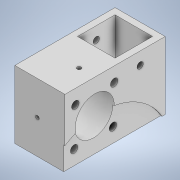
# Autodesk Inventor part: nema_mount
Saved by Autodesk Inventor 2022.3 (Build 263350000, 350)
## iProperties
Created: 2022-06-10
Part Number: nema_mount
Material: Generic
Document SubType Name: Modeling
Designer: Martijn
Density: 1 g/cm^3
Appearance: Default
Author: Martijn
Autodesk Inventor part; units mm, degrees
ref_plane "YZ Plane" through (0, 0, 0) normal (1, 0, 0) x (0, 1, 0)
ref_plane "XZ Plane" through (0, 0, 0) normal (0, 1, 0) x (-1, 0, 0)
ref_plane "XY Plane" through (0, 0, 0) normal (0, 0, 1) x (1, 0, 0)
sketch "Sketch1" plane through (0, 0, 0) normal (0, 0, 1) x (1, 0, 0)
  line L0 (0, 0) -> (40, 0)
  line L1 (40, 0) -> (40, 54)
  line L2 (40, 54) -> (0, 54)
  line L3 (0, 54) -> (0, 0)
  dimension "d0" = 40
  dimension "d1" = 54
  constraints: 8 end point, 2 parallel, 1 horizontal, 1 perpendicular
  measures "d0" distance of L0.start L0.end
  measures "d1" distance of L2.end L0.start
extrude "Extrusion1" add sketch "Sketch1" along normal blind 80
sketch "Sketch3" plane through (0, 0, 0) normal (0, -1, 0) x (1, 0, 0)
  line L0 (5, 5) -> (35, 5)
  line L1 (35, 5) -> (35, 35)
  line L2 (35, 35) -> (5, 35)
  line L3 (5, 35) -> (5, 5)
  line L4 (0, 0) -> (40, 0) projected
  line L5 (0, 0) -> (0, 80) projected
  dimension "d7" = 30
  dimension "d8" = 30
  dimension "d9" = 5
  dimension "d10" = 5
  constraints: 8 end point, 2 parallel, 1 horizontal, 1 perpendicular
  measures "d7" distance between parallel lines of L2 L0
  measures "d8" distance between parallel lines of L1 L3
  measures "d9" distance between parallel lines of L4 L0
  measures "d10" distance between parallel lines of L5 L3
extrude "Extrusion2" cut sketch "Sketch3" against normal blind 80
sketch "Sketch4" plane through (0, 0, 0) normal (-1, 0, 0) x (0, 0, 1)
  line L0 (35, 0) -> (35, 54) projected
  line L1 (35, 5.8) -> (77.4, 5.8)
  line L2 (77.4, 5.8) -> (77.4, 48.2)
  line L3 (77.4, 48.2) -> (35, 48.2)
  line L4 (35, 48.2) -> (35, 5.8)
  line L5 (0, 0) -> (80, 0) projected
  dimension "d13" = 42.4
  dimension "d14" = 42.4
  dimension "d15" = 5.8
  constraints: 8 end point, 2 parallel, 1 horizontal, 1 perpendicular, 1 point on line
  measures "d13" distance between parallel lines of L3 L1
  measures "d14" distance between parallel lines of L0 L2
  measures "d15" distance between parallel lines of L5 L1
extrude "Extrusion3" cut sketch "Sketch4" against normal blind 9
sketch "Sketch5" plane through (9, 0, 0) normal (-1, 0, 0) x (0, 0, 1)
  circle A0 centre (71.7, 42.5) radius 1.6
  circle A1 centre (71.7, 11.5) radius 1.6
  circle A2 centre (40.7, 42.5) radius 1.6
  circle A3 centre (40.7, 11.5) radius 1.6
  circle A4 centre (56.2, 27) radius 2.75
  line L0 (71.7, 42.5) -> (71.7, 11.5)
  line L1 (71.7, 11.5) -> (40.7, 11.5)
  line L2 (40.7, 11.5) -> (40.7, 42.5)
  line L3 (40.7, 42.5) -> (71.7, 42.5)
  line L4 (77.4, 48.2) -> (77.4, 5.8) projected
  line L5 (35, 48.2) -> (77.4, 48.2) projected
  point P0 (0, 0)
  dimension "d18" = 3.2
  dimension "d19" = 31
  dimension "d20" = 31
  dimension "d21" = 5.7
  dimension "d22" = 5.7
  dimension "d23" = 15.5
  dimension "d24" = 15.5
  dimension "d25" = 5.5
  constraints: 8 end point, 5 centre point, 3 equal radius, 3 perpendicular, 1 vertical
  measures "d18" diameter of A0
  measures "d19" distance of L0.start L0.end
  measures "d20" distance of L2.end L0.start
  measures "d21" distance between parallel lines of L4 L0
  measures "d22" distance between parallel lines of L5 L3
  measures "d23" horizontal distance of A4.centre L0.start
  measures "d24" horizontal distance of L2.end A4.centre
  measures "d25" diameter of A4
extrude "Extrusion4" cut sketch "Sketch5" against normal blind 40 contours A0 L0 L3 | L3 L0 A0 | L3 L2 A2 | A2 L2 L3 | L0 L1 A1 | A1 L1 L0 | L2 L1 A3 | A3 L1 L2 | A4
sketch "Sketch7" plane through (40, 0, 0) normal (1, 0, 0) x (0, 0, -1)
  circle A0 centre (-56.2, 27) radius 15.5
  circle A1 centre (-56.2, 27) radius 2.75 projected
  circle A2 centre (-71.7, 11.5) radius 1.6 projected
  circle A3 centre (-71.7, 11.5) radius 3
  circle A4 centre (-40.7, 11.5) radius 1.6 projected
  circle A5 centre (-40.7, 11.5) radius 3
  circle A6 centre (-40.7, 42.5) radius 1.6 projected
  circle A7 centre (-40.7, 42.5) radius 3
  circle A8 centre (-71.7, 42.5) radius 1.6 projected
  circle A9 centre (-71.7, 42.5) radius 3
  point P0 (0, 0)
  point P1 (-72.8896, 14.2541)
  point P2 (-68.9459, 10.3104)
  point P3 (-43.4541, 10.3104)
  point P4 (-39.5104, 14.2541)
  point P5 (-39.5104, 39.7459)
  point P6 (-43.4541, 43.6896)
  point P7 (-68.9459, 43.6896)
  point P8 (-72.8896, 39.7459)
  dimension "d28" = 31
  dimension "d29" = 6
  constraints: 5 centre point, 4 coincident, 3 equal radius, 1 concentric
  measures "d28" diameter of A0
  measures "d29" diameter of A3
extrude "Extrusion5" cut sketch "Sketch7" against normal blind 25 contours A0 | A2 | A3 | A4 | A5 | A6 | A7 | A8 | A9
sketch "Sketch8" plane through (0, 0, 80) normal (0, 0, 1) x (1, 0, 0)
  circle A0 centre (18, 27) radius 1.5
  line L0 (40, 54) -> (0, 54) projected
  line L1 (40, 0) -> (40, 54) projected
  line L2 (15, 24.25) -> (15, 29.75) projected
  point P0 (0, 0)
  dimension "d32" = 3
  dimension "d33" = 27
  dimension "d35" = 3
  constraints: 1 centre point
  measures "d32" diameter of A0
  measures "d33" distance from line of L0 A0.centre
  measures "d35" distance from line of L2 A0.centre
extrude "Extrusion6" cut sketch "Sketch8" against normal blind 10
sketch "Sketch9" plane through (0, 54, 0) normal (0, 1, 0) x (1, 0, 0)
  circle A0 centre (27.5, -56.2) radius 1.6
  line L0 (15, -58.95) -> (15, -53.45) projected
  line L1 (35, -35) -> (5, -35) projected
  point P0 (0, 0)
  dimension "d38" = 12.5
  dimension "d39" = 3.2
  dimension "d43" = 21.2
  constraints: 1 centre point
  measures "d38" distance from line of A0.centre L0
  measures "d39" diameter of A0
  measures "d43" distance from line of L1 A0.centre
extrude "Extrusion7" cut sketch "Sketch9" against normal blind 20
sketch "Sketch10" plane through (40, 0, 0) normal (1, 0, 0) x (0, 0, -1)
  circle A0 centre (-50, -27.6494) radius 55
  circle A1 centre (-56.2, 27) radius 2.75 projected
  line L0 (-80, 0) -> (-80, 54) projected
  point P0 (0, 0)
  point P1 (-58.9239, 26.6218)
  point P2 (-53.4606, 27.2416)
  point P3 (-35, 54)
  dimension "d44" = 110
  dimension "d48" = 55
  dimension "d49" = 15
  constraints: 1 centre point
  measures "d44" diameter of A0
  measures "d48" distance of A1.centre A0.centre
  measures "d49" horizontal distance of point (-35, 54) A0.centre
extrude "Extrusion8" cut sketch "Sketch10" against normal blind 1 contours A0 A1 picked at (-46.0473, -46.3669)
sketch "Sketch11" plane through (9, 0, 0) normal (-1, 0, 0) x (0, 0, 1)
  circle A0 centre (56.2, 27) radius 11.2
  circle A1 centre (56.2, 27) radius 2.75 projected
  point P0 (0, 0)
  dimension "d50" = 22.4
  constraints: 1 centre point, 1 concentric
  measures "d50" diameter of A0
extrude "Extrusion9" cut sketch "Sketch11" against normal blind 2.2
sketch "Sketch12" plane through (40, 0, 0) normal (1, 0, 0) x (0, 0, -1)
  circle A0 centre (-20, 44) radius 2.5
  line L0 (0, 54) -> (-80, 54) projected
  point P0 (0, 0)
  point P1 (-5, 54)
  dimension "d53" = 15
  dimension "d54" = 5
  dimension "d55" = 10
  constraints: 1 centre point
  measures "d53" horizontal distance of point (-5, 54) A0.centre
  measures "d54" diameter of A0
  measures "d55" distance from line of L0 A0.centre
extrude "Extrusion10" cut sketch "Sketch12" against normal blind 10
sketch "Sketch13" plane through (0, 0, 0) normal (-1, 0, 0) x (0, 0, 1)
  circle A0 centre (20, 44) radius 2.5 projected
  circle A1 centre (20, 44) radius 2.5
  circle A2 centre (20, 10) radius 2.5
  line L0 (0, 54) -> (80, 54) projected
  line L1 (0, 0) -> (80, 0) projected
  point P0 (5, 54)
  dimension "d58" = 15
  dimension "d59" = 15
  dimension "d62" = 5
  dimension "d63" = 10
  constraints: 2 centre point, 1 coincident
  measures "d58" horizontal distance of point (5, 54) A1.centre
  measures "d59" horizontal distance of point (5, 54) A2.centre
  measures "d62" diameter of A2
  measures "d63" distance from line of L1 A2.centre
extrude "Extrusion11" cut sketch "Sketch13" against normal blind 10
equation "\"d22\" = d21"
body "Solid1"
